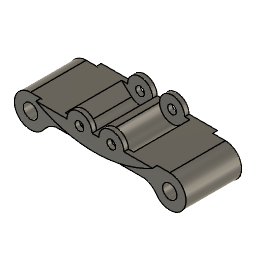
cap_adapter (Autodesk Fusion 360 design; units mm, degrees)
Autodesk Fusion 360 part; units mm, degrees
note: some values were not read from the file. Set by a fixed rule: which sketch regions a step uses.
sketch "Sketch1" plane through (0, 0, 0) normal (0, 1, 0) x (1, 0, 0)
  circle A0 centre (8.5, -5.3702) radius 3.125
  line L0 (8.5, -5.3702) -> (69.5, -5.3702) construction
  circle A1 centre (69.5, -5.3702) radius 3.125
  line L1 (8.5, -5.3702) -> (8.5, -4.8202)
  line L2 (69.5, -5.3702) -> (69.5, -4.8202)
  line L3 (8.5, -4.8202) -> (69.5, -4.8202)
  circle A2 centre (32, -12.4952) radius 1.9
  circle A3 centre (32, -12.4952) radius 3.8
  circle A4 centre (32, -12.4952) radius 5.5
  circle A5 centre (46, -12.4952) radius 3.8
  circle A6 centre (46, -12.4952) radius 5.5
  circle A7 centre (46, -12.4952) radius 1.9
  line L4 (8.5, -5.3702) -> (8.5, 0.4006) construction
  line L5 (32, -12.4952) -> (28.2807, -8.4434) construction
  circle A8 centre (8.5, -5.3702) radius 7.125
  circle A9 centre (69.5, -5.3702) radius 7.125
  line L6 (8.5, -5.3702) -> (8.5, -12.4952) construction
  line L7 (69.5, -5.3702) -> (69.5, -12.4952) construction
  line L8 (8.5, -12.4952) -> (69.5, -12.4952)
  line L9 (39, -4.8202) -> (39, -12.4952) construction
  line L10 (11.5762, -4.8202) -> (19.5894, -4.8202)
  line L11 (66.4238, -4.8202) -> (58.4302, -4.8202)
  line L12 (8.5, -4.8202) -> (14.4185, -1.4032) construction
  line L13 (69.5, -4.8202) -> (63.5815, -1.4032) construction
  arc A10 (58.4302, -4.8202) -> (63.5815, -1.4032) centre (56.9033, 3.0731) ccw
  arc A11 (14.4185, -1.4032) -> (19.5894, -4.8202) centre (21.0864, 3.0662) ccw
  line L14 (46, -12.4952) -> (49.8903, -8.6074) construction
  line L15 (28.2807, -8.4434) -> (23.8667, -12.4952)
  line L16 (49.8903, -8.6074) -> (53.7757, -12.4952)
  line L17 (39, -4.8202) -> (39, -5.8202)
  line L18 (69.5, -12.4952) -> (64.0042, -12.4952)
  line L19 (8.5, -12.4952) -> (12.9956, -12.4952)
  arc A12 (64.0042, -12.4952) -> (12.9956, -12.4952) centre (38.4999, -57.8632) ccw
  point P0 (64.0042, -12.4952)
  point P1 (12.9956, -12.4952)
  dimension "d1" = 6.25
  dimension "d2" = 61
  dimension "d3" = 6.25
  dimension "d6" = 0.55
  dimension "d7" = 0.55
  dimension "d8" = 3.8
  dimension "d9" = 7.6
  dimension "d10" = 11
  dimension "d11" = 3.8
  dimension "d12" = 7.6
  dimension "d13" = 11
  dimension "d27" = 14.25
  dimension "d28" = 14.25
  dimension "d29" = 14
  dimension "d30" = 7
  dimension "d31" = 7.675
  dimension "d37" = 1
  constraint coincident A0.centre L0.start
  constraint horizontal L0
  constraint coincident L0.end A1.centre
  constraint perpendicular L0 L1
  constraint perpendicular L0 L2
  constraint concentric A2 A3
  constraint concentric A3 A4
  constraint concentric A5 A7
  constraint concentric A5 A6
  constraint perpendicular L0 L4
  constraint coincident A2.centre A3.centre
  constraint coincident A4 L5.end
  constraint concentric A0 A8
  constraint concentric A1 A9
  constraint coincident A8 L6.end
  constraint perpendicular L0 L6
  constraint coincident A9 L7.end
  constraint perpendicular L0 L7
  constraint midpoint L3 L9.start
  constraint midpoint L8 L9.end
  constraint coincident A5.centre L8
  constraint coincident L3 L10.start
  constraint coincident A0 L10.start
  constraint parallel L3 L10
  constraint coincident A1 L11.start
  constraint coincident L3 L11.start
  constraint parallel L3 L11
  constraint coincident A8 L12.end
  constraint coincident A9 L13.end
  constraint tangent A9 A10
  constraint tangent A8 A11
  constraint coincident A5.centre A6.centre
  constraint coincident A6 L14.end
  constraint coincident L8 L15.end
  constraint tangent A4 L15
  constraint coincident L8 L16.end
  constraint tangent A6 L16
  constraint perpendicular L0 L17
  constraint coincident L8 P0
  constraint coincident P0 L18.end
  constraint coincident L8 P1
  constraint coincident P1 L19.end
  constraint coincident L17.end A12
  measures "d1" diameter of A0
  measures "d2" distance of A0.centre L0.end
  measures "d3" diameter of A1
  measures "d6" distance of A0.centre L1.end
  measures "d7" distance of L0.end L2.end
  measures "d8" diameter of A2
  measures "d9" diameter of A3
  measures "d10" diameter of A4
  measures "d11" diameter of A7
  measures "d12" diameter of A5
  measures "d13" diameter of A6
  measures "d27" diameter of A8
  measures "d28" diameter of A9
  measures "d29" horizontal distance of A2.centre A5.centre
  measures "d30" distance of A2.centre L9
  measures "d31" distance of L3 A2.centre
  measures "d37" distance of L9.start L17.end
extrude "Extrude4" add sketch "Sketch1" along normal blind 24.4 contours L3 A8 L8 L10 L17 L19 A12 | L3 A8 L10 A11 | L3 A9 L8 L11 L17 L18 A12 | A8 | L3 A9 L11 A10 | A4 A6 L8 L15 L16 A12 | A9
extrude "Extrude9" add sketch "Sketch1" against normal blind 2.1 contours A4 A6 L8 L15 L16 A12
extrude "Extrude10" add sketch "Sketch1" against normal blind 2 from surface at -0.1 contours A6 L8 L16 | A4 L8 L15 | A5 A6 L8 | A5 A6 L8 | A3 A4 L8 | A3 A4 L8 | A5 A7 L8 | A5 A7 L8 | A2 A3 L8 | A2 A3 L8
extrude "Extrude11" add sketch "Sketch1" along normal blind 2.1 from surface at 24.4 contours A4 A6 L8 L15 L16 A12
extrude "Extrude12" add sketch "Sketch1" along normal blind 2 from surface at 24.5 contours A6 L8 L16 | A4 L8 L15 | A5 A6 L8 | A5 A6 L8 | A3 A4 L8 | A3 A4 L8 | A5 A7 L8 | A5 A7 L8 | A2 A3 L8 | A2 A3 L8
extrude "Extrude5" [suppressed]
extrude "Extrude6" [suppressed]
extrude "Extrude7" [suppressed]
extrude "Extrude8" [suppressed]
component "cap_adapter v8" placed x (1, 0, 0) y (0, 1, 0) z (0, 0, 1) at (0, 0, 0)
